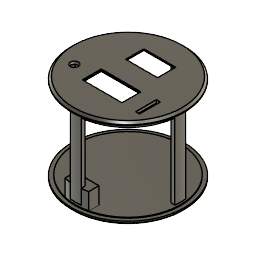
ESP32-Thermostat (Autodesk Fusion 360 design; units mm, degrees)
Autodesk Fusion 360 part; units mm, degrees
note: some values were not read from the file. Set by a fixed rule: which face or edge a step refers to.
sketch "Sketch1" plane through (0, 0, 0) normal (0, 0, 1) x (1, 0, 0)
  circle A0 centre (30, 30) radius 36.35
  circle A1 centre (30, 30) radius 39
  line L0 (30, 30) -> (25.9234, -8.7864)
  line L1 (30, 30) -> (69, 30) construction
  line L2 (30, 30) -> (34.0766, -8.7864)
  line L3 (30, 30) -> (69, 30) construction
  circle A2 centre (30, 30) radius 33.35
  dimension "d1" = 72.7
  dimension "d2" = 78
  dimension "d39" = 96
  dimension "d40" = 84
  dimension "d41" = 66.7
  constraint concentric A0 A1
  constraint horizontal L1
  constraint coincident A0.centre A1.centre
  constraint horizontal L3
  constraint concentric A1 A2
  measures "d1" diameter of A0
  measures "d2" diameter of A1
  measures "d39" angle of L0 L1
  measures "d40" angle of L2 L3
  measures "d41" diameter of A2
extrude "Extrude4" add sketch "Sketch1" along normal blind 2 and the other way blind 3 thin wall 3 inside contours A0 L0 L2 A2 | A0 L0 L2 A2 | L0 L2 A2 | L0 L2 A2 makes body 1
extrude "Extrude5" add sketch "Sketch1" against normal blind 2 from surface at 2 bodies 1
chamfer "Chamfer1" distance 1.5 angle 45 1 edges at (-6.3608, 44.103, 2) on bodies 1
sketch "Sketch2" plane through (0, 0, 2) normal (0, 0, 1) x (-1, 0, 0)
  circle A0 centre (-30, -30) radius 37.5
  line L0 (-41, -39.4685) -> (-19, -39.4685)
  line L1 (-19, -39.4685) -> (-19, -51.9685)
  line L2 (-19, -51.9685) -> (-41, -51.9685)
  line L3 (-41, -51.9685) -> (-41, -39.4685)
  line L4 (-41, -39.4685) -> (-19, -51.9685) construction
  line L5 (-19, -39.4685) -> (-41, -51.9685) construction
  circle A1 centre (-4.1687, -18.6626) radius 2.75
  line L6 (-43.2, -12.6626) -> (-16.8, -12.6626)
  line L7 (-16.8, -12.6626) -> (-16.8, -24.6626)
  line L8 (-16.8, -24.6626) -> (-43.2, -24.6626)
  line L9 (-43.2, -24.6626) -> (-43.2, -12.6626)
  line L10 (-43.2, -12.6626) -> (-16.8, -24.6626) construction
  line L11 (-16.8, -12.6626) -> (-43.2, -24.6626) construction
  line L12 (-56.5231, -11.5626) -> (-53.8231, -11.5626)
  line L13 (-53.8231, -11.5626) -> (-53.8231, -25.7626)
  line L14 (-53.8231, -25.7626) -> (-56.5231, -25.7626)
  line L15 (-56.5231, -25.7626) -> (-56.5231, -11.5626)
  line L16 (-56.5231, -11.5626) -> (-53.8231, -25.7626) construction
  line L17 (-53.8231, -11.5626) -> (-56.5231, -25.7626) construction
  line L18 (-50.5, -11.6626) -> (-9.5, -11.6626)
  line L19 (-9.5, -11.6626) -> (-9.5, -25.6626)
  line L20 (-9.5, -25.6626) -> (-50.5, -25.6626)
  line L21 (-50.5, -25.6626) -> (-50.5, -11.6626)
  line L22 (-50.5, -11.6626) -> (-9.5, -25.6626) construction
  line L23 (-9.5, -11.6626) -> (-50.5, -25.6626) construction
  point P0 (-30, -45.7185)
  point P1 (-30, -18.6626)
  point P2 (-55.1731, -18.6626)
  point P3 (-30, -18.6626)
  point P4 (-30, -30)
  dimension "d23" = 22
  dimension "d24" = 12.5
  dimension "d25" = 5.5
  dimension "d28" = 26.4
  dimension "d29" = 12
  dimension "d30" = 2.7
  dimension "d31" = 14.2
  dimension "d34" = 41
  dimension "d35" = 14
  constraint horizontal L0
  constraint perpendicular L0 L1
  constraint parallel L0 L2
  constraint parallel L1 L3
  constraint coincident L4 P0
  constraint coincident L5 P0
  constraint horizontal L6
  constraint perpendicular L6 L7
  constraint parallel L6 L8
  constraint parallel L7 L9
  constraint coincident L10 P3
  constraint coincident L11 P3
  constraint horizontal L12
  constraint perpendicular L12 L13
  constraint parallel L12 L14
  constraint parallel L13 L15
  constraint coincident L16 P2
  constraint coincident L17 P2
  constraint horizontal L18
  constraint perpendicular L18 L19
  constraint parallel L18 L20
  constraint parallel L19 L21
  constraint coincident L22 P3
  constraint coincident L23 P3
  constraint coincident P3 P1
  constraint horizontal A1.centre P3
  constraint horizontal P3 P2
  constraint coincident P4 A0.centre
  constraint vertical P3 P4
  constraint vertical P0 P4
  measures "d23" distance of L1.end L2.end
  measures "d24" distance of L0.end L1.end
  measures "d25" diameter of A1
  measures "d28" distance of L7.end L8.end
  measures "d29" distance of L6.end L7.end
  measures "d30" distance of L13.end L14.end
  measures "d31" distance of L12.end L13.end
  measures "d34" distance of L19.end L20.end
  measures "d35" distance of L18.end L19.end
extrude "Extrude6" cut sketch "Sketch2" against normal up to surface (2 mm away) contours L0 L1 L2 L3 | A1 bodies 1
extrude "Extrude7" cut sketch "Sketch2" against normal up to surface (2 mm away) contours L6 L7 L8 L9 | L12 L13 L14 L15 bodies 1
extrude "Extrude8" cut sketch "Sketch2" along normal blind 1 from surface at -2 contours L18 L19 L20 L21 bodies 1
extrude "Extrude9" add sketch "Sketch1" against normal blind 55.3 contours A0 L0 L2 A2 picked at (27.9226, -5.2695) bodies 1
sketch "Sketch3" plane through (0, 0, -55.3) normal (0, 0, -1) x (1, 0, 0)
  arc A0 (33.7996, 6.1509) -> (26.2004, 6.1509) centre (30, -30) ccw
  line L0 (26.2004, 6.1509) -> (26.514, 3.1673)
  arc A1 (33.486, 3.1673) -> (26.514, 3.1673) centre (30, -30) ccw
  line L1 (33.486, 3.1673) -> (33.7996, 6.1509)
  circle A2 centre (29.9807, 4.7934) radius 1
  dimension "d46" = 2
  measures "d46" diameter of A2
extrude "Extrude10" cut sketch "Sketch3" against normal blind 8 contours A2 bodies 1
pattern_circular "C-Pattern2" count 4 over 360 about axis through (30, 30, -0.4) along (0, 0, 1) of "Extrude9", "Extrude10"
chamfer "Chamfer2" distance 1 angle 45 4 edges at (30, 51.9685, 0) (41, 45.7185, 0) (30, 39.4685, 0) (19, 45.7185, 0) on bodies 1
chamfer "Chamfer3" distance 0.5 angle 45 4 edges at (30, 12.6626, 2) (43.2, 18.6626, 2) (30, 24.6626, 2) (16.8, 18.6626, 2) on bodies 1
extrude "Extrude11" add sketch "Sketch1" against normal blind 3 from surface at -57.3 separate body makes body 2
extrude "Extrude17" add sketch "Sketch1" along normal blind 0.5 from surface at -57.3 contours A0 L0 L2 A2 | A0 L0 L2 A2 | L0 L2 A2 | L0 L2 A2 bodies 2
extrude "Extrude12" [suppressed]
move_face "OffsetFaces1" [suppressed]
sketch "Sketch4" plane through (0, 0, -55.3) normal (0, 0, -1) x (1, 0, 0)
  arc A0 (33.7996, 6.1509) -> (26.2004, 6.1509) centre (30, -30) ccw
  line L0 (33.486, 3.1673) -> (33.7996, 6.1509)
  arc A1 (33.486, 3.1673) -> (26.514, 3.1673) centre (30, -30) ccw
  circle A2 centre (29.9807, 4.7934) radius 1
  line L1 (26.2004, 6.1509) -> (26.514, 3.1673)
  circle A3 centre (30, -30) radius 36.35
  circle A4 centre (30, -30) radius 33.35
  line L2 (30, -30) -> (22.4979, 2.4952)
  line L3 (30, -30) -> (63.35, -30) construction
  line L4 (22.4979, 2.4952) -> (21.823, 5.4184)
  line L5 (30, -30) -> (38.0858, 5.0233)
  line L6 (30, -30) -> (66.0791, -30) construction
  line L7 (38.0858, 5.0233) -> (38.177, 5.4184)
  line L8 (21.823, 8.2782) -> (38.177, 8.2782)
  line L9 (38.177, 8.2782) -> (38.177, -1.7218)
  line L10 (38.177, -1.7218) -> (21.823, -1.7218)
  line L11 (21.823, -1.7218) -> (21.823, 8.2782)
  circle A5 centre (30, 2.35) radius 1.5
  dimension "d60" = 103
  dimension "d61" = 77
  dimension "d62" = 10
  dimension "d67" = 3
  constraint concentric A1 A3
  constraint concentric A0 A4
  constraint coincident A1.end A4
  constraint horizontal L3
  constraint coincident A0.centre A1.centre
  constraint coincident A3 L4.end
  constraint parallel L2 L4
  constraint horizontal L6
  constraint coincident A3 L7.end
  constraint parallel L5 L7
  constraint horizontal L8
  constraint vertical L9
  constraint horizontal L10
  constraint vertical L11
  measures "d60" angle of L2 L3
  measures "d61" angle of L5 L6
  measures "d62" distance of L8.start L10.end
  measures "d67" diameter of A5
extrude "Extrude13" add sketch "Sketch4" against normal blind 10 separate body contours L0 A3 A4 L5 L7 | L1 A3 A4 L4 | A1 A4 L2 L5 L10 A5 | A4 L5 L7 L9 | A4 L4 L11 | A1 A4 A5 | A4 L5 L9 L10 | A4 L2 L10 L11 makes body 3
extrude "Extrude14" add sketch "Sketch4" along normal blind 2 contours A0 L0 A1 A2 L1 A3 A4 A5 | L0 A3 A4 L5 L7 | L1 A3 A4 L4 | A1 A4 L2 L5 L10 A5 | A4 L5 L7 L9 | A4 L4 L11 | A1 A4 A5 | A1 A2 A4 A5 | A4 L5 L9 L10 | A4 L2 L10 L11 | A2 A5 | A2 A5 bodies 3
extrude "Extrude15" cut sketch "Sketch4" along normal blind -6 and the other way up to surface (-2 mm away) contours A1 A4 A5 | A1 A2 A4 A5 | A2 A5 picked at (29.9883, 3.8294) bodies 3
extrude "Extrude16" cut sketch "Sketch4" along normal up to surface (3.5 mm away) from surface at 1.5 contours A1 A4 A5 | A1 A2 A4 A5 | A2 A5 picked at (29.9883, 3.8294) bodies 2
chamfer "Chamfer4" distance 2 angle 45 1 edges at (28.6015, -2.8924, -60.3) on bodies 2
pattern_circular "C-Pattern3" count 4 over 360 about axis through (30, 30, -0.4) along (0, 0, 1) of 2 faces at (32.2399, -4.4283, -59.8556) (31.4925, -2.4994, -57.8) on bodies 2
chamfer "Chamfer5" distance 2 angle 45 1 edges at (-6.3608, 44.103, -60.3) on bodies 2
chamfer "Chamfer6" distance 1 angle 45 1 edges at (-4.4961, 16.6202, -60.3) on bodies 2
equation "d41 = 72.700 mm - 6 * 1 mm"
equation "d42 = -61.3 mm + 6 mm"
named bodies: "Face", "Cover", "adapter"
